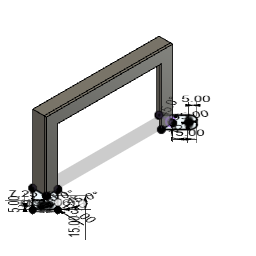
Halterung Sync-Box v2 (Autodesk Fusion 360 design; units mm, degrees)
Autodesk Fusion 360 part; units mm, degrees
sketch "Skizze1" plane through (0, 0, 0) normal (1, 0, 0) x (0, 0, -1)
  line L0 (-44.2076, 32.5954) -> (62.7924, 32.5954)
  line L1 (-44.2076, 32.5954) -> (-44.2076, -25.4046)
  line L2 (62.7924, 32.5954) -> (62.7924, -25.4046)
  line L3 (-44.2076, -25.4046) -> (-46.2076, -25.4046)
  line L4 (-46.2076, -25.4046) -> (-46.2076, 34.5954)
  line L5 (-46.2076, 34.5954) -> (64.7924, 34.5954)
  line L6 (64.7924, 34.5954) -> (64.7924, -25.4046)
  line L7 (62.7924, -25.4046) -> (64.7924, -25.4046)
  dimension "d1" = 107
  dimension "d2" = 58
  dimension "d3" = 58
  dimension "d4" = 2
  dimension "d5" = 60
  dimension "d6" = 111
  dimension "d7" = 60
  constraint horizontal L0
  constraint perpendicular L0 L1
  constraint perpendicular L0 L2
  constraint perpendicular L1 L3
  constraint perpendicular L3 L4
  constraint perpendicular L4 L5
  constraint perpendicular L0 L6
  measures "d1" distance of L0.start L0.end
  measures "d2" distance of L0.start L1.end
  measures "d3" distance of L0.end L2.end
  measures "d4" distance of L1.end L3.end
  measures "d5" distance of L3.end L4.end
  measures "d6" distance of L4.end L5.end
  measures "d7" distance of L5.end L6.end
extrude "Extrusion1" add sketch "Skizze1" along normal blind 10 makes body 1
sketch "Skizze2" plane through (10, 0, 0) normal (1, 0, 0) x (0, 0, -1)
  line L0 (-44.2076, 32.5954) -> (62.7924, 32.5954)
  line L1 (62.7924, 32.5954) -> (62.7924, -25.4046)
  line L2 (62.7924, -25.4046) -> (64.7924, -25.4046)
  line L3 (64.7924, -25.4046) -> (64.7924, 34.5954)
  line L4 (64.7924, 34.5954) -> (-46.2076, 34.5954)
  line L5 (-46.2076, 34.5954) -> (-46.2076, -25.4046)
  line L6 (-46.2076, -25.4046) -> (-44.2076, -25.4046)
  line L7 (-44.2076, -25.4046) -> (-44.2076, 32.5954)
  line L8 (-46.2076, 34.5954) -> (64.7924, 34.5954)
  line L9 (64.7924, 34.5954) -> (64.7924, 24.5954)
  line L10 (64.7924, 24.5954) -> (-46.2076, 24.5954)
  line L11 (-46.2076, 24.5954) -> (-46.2076, 34.5954)
  line L12 (-46.2076, -25.4046) -> (-36.2076, -25.4046)
  line L13 (-36.2076, -25.4046) -> (-36.2076, 24.5954)
  line L14 (-36.2076, 24.5954) -> (-46.2076, 24.5954)
  line L15 (-46.2076, 24.5954) -> (-46.2076, -25.4046)
  line L16 (64.7924, -25.4046) -> (54.7924, -25.4046)
  line L17 (54.7924, -25.4046) -> (54.7924, 24.5954)
  line L18 (54.7924, 24.5954) -> (64.7924, 24.5954)
  line L19 (64.7924, 24.5954) -> (64.7924, -25.4046)
  dimension "d10" = 10
  dimension "d11" = 10
  dimension "d12" = 10
  constraint horizontal L8
  constraint vertical L9
  constraint horizontal L10
  constraint vertical L11
  constraint coincident L4.end L5.start
  constraint horizontal L12
  constraint vertical L13
  constraint horizontal L14
  constraint vertical L15
  constraint coincident L5.end L6.start
  constraint horizontal L16
  constraint vertical L17
  constraint horizontal L18
  constraint vertical L19
  constraint coincident L2.end L3.start
  measures "d10" distance of L4.end L10.end
  measures "d11" distance of L5.end L12.end
  measures "d12" distance of L2.end L16.end
extrude "Extrusion2" add sketch "Skizze2" along normal blind 2 separate body makes body 2
ref_plane "Arbeitsebene2" through (5, -25.4046, 45.2076) normal (0, -1, 0) x (0, 0, -1)
sketch "Skizze4" plane through (5, -25.4046, 45.2076) normal (0, -1, 0) x (1, 0, 0)
  line L0 (-5, 1) -> (8.0711, 14.0711)
  line L1 (-5, 1) -> (17.1415, 1) construction
  line L2 (7, -9) -> (19.0711, 3.0711)
  line L3 (7, -9) -> (28.7493, -9) construction
  line L4 (19.0711, 10.1421) -> (15.1421, 14.0711)
  circle A0 centre (13.1976, 8.9445) radius 2.5
  line L5 (7, -100) -> (19.0711, -112.0711)
  line L6 (19.0711, -119.1421) -> (15.1421, -123.0711)
  line L7 (8.0711, -123.0711) -> (-5, -110)
  line L8 (-5, -110) -> (5, -110)
  circle A1 centre (13.591, -117.5511) radius 2.5
  line L9 (-5, -110) -> (7, -110)
  line L10 (7, -110) -> (7, -100)
  line L11 (-5, 1) -> (7, 1)
  line L12 (7, 1) -> (7, -9)
  arc A2 (19.0711, 3.0711) -> (19.0711, 10.1421) centre (15.5355, 6.6066) ccw
  arc A3 (15.1421, 14.0711) -> (8.0711, 14.0711) centre (11.6066, 10.5355) ccw
  arc A4 (19.0711, -119.1421) -> (19.0711, -112.0711) centre (15.5355, -115.6066) ccw
  arc A5 (8.0711, -123.0711) -> (15.1421, -123.0711) centre (11.6066, -119.5355) ccw
  point P0 (11.6066, 17.6066)
  point P1 (22.6066, 6.6066)
  point P2 (7, 1)
  point P3 (-5, 1)
  point P4 (7, -9)
  point P5 (-5, -110)
  point P6 (7, -100)
  point P7 (7, -110)
  dimension "d18" = 45
  dimension "d19" = 45
  dimension "d20" = 15
  dimension "d21" = 5
  dimension "d23" = 15.5563
  dimension "d24" = 7.25
  dimension "d25" = 5
  dimension "d26" = 45
  dimension "d27" = 15
  dimension "d28" = 5
  dimension "d29" = 7.75
  dimension "d30" = 5
  dimension "d33" = 5
  constraint horizontal L1
  constraint horizontal L3
  constraint perpendicular L2 L4
  constraint coincident P3 L0.start
  constraint coincident L2.start L3.start
  constraint perpendicular L5 L6
  constraint perpendicular L6 L7
  constraint coincident P5 L7.end
  constraint coincident P6 L5.start
  constraint coincident P7 L9.end
  constraint coincident P2 L11.end
  constraint coincident P4 L2.start
  constraint coincident P1 L2
  constraint coincident P1 L4
  constraint tangent L2 A2
  constraint tangent L4 A2
  constraint coincident P0 L0
  constraint coincident P0 L4
  constraint tangent L0 A3
  constraint tangent L4 A3
  constraint equal A2 A3
  constraint tangent L5 A4
  constraint tangent L6 A4
  constraint equal A2 A4
  constraint tangent L6 A5
  constraint tangent L7 A5
  constraint equal A2 A5
  measures "d18" angle of L0 L1
  measures "d19" angle of L2 L3
  measures "d20" distance of L4 P2
  measures "d21" diameter of A0
  measures "d23" distance of P0 P1
  measures "d24" distance of L0 A0.centre
  measures "d25" distance of L4 A0.centre
  measures "d26" angle of L7 L8
  measures "d27" distance of L6 P7
  measures "d28" diameter of A1
  measures "d29" distance of L5 A1.centre
  measures "d30" distance of L6 A1.centre
  measures "d33" radius of A2
extrude "Extrusion3" [suppressed]
fillet "Abrundung1" [suppressed]
fillet "Abrundung2" [suppressed]
